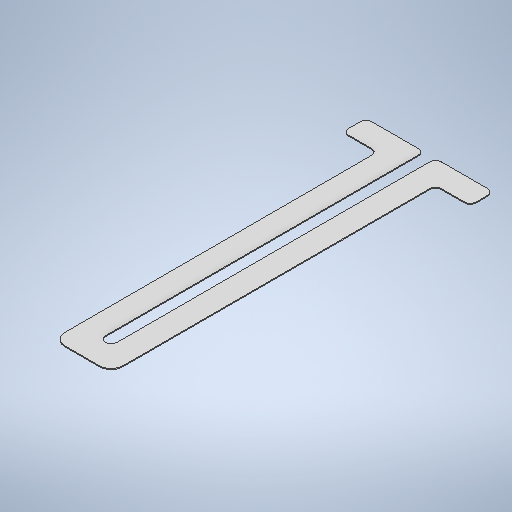
# Autodesk Inventor part: Medio
Saved by Autodesk Inventor 2025.4 (Build 294407000, 407)
## iProperties
Created: 2026-04-15
Part Number: Medio
Material: Generic
Document SubType Name: Modeling
Designer: gdira
Density: 1 g/cm^3
Appearance: Default
Author: gdira
Autodesk Inventor part; units mm, degrees
ref_plane "YZ Plane" through (0, 0, 0) normal (1, 0, 0) x (0, 1, 0)
ref_plane "XZ Plane" through (0, 0, 0) normal (0, 1, 0) x (-1, 0, 0)
ref_plane "XY Plane" through (0, 0, 0) normal (0, 0, 1) x (1, 0, 0)
sketch "Sketch1" plane through (0, 0, 0) normal (0, 1, 0) x (-1, 0, 0)
  line L0 (1.2188, -16.0155) -> (-0.7718, -16.0155)
  line L1 (-4.7718, -16.0123) -> (-12.7718, -16.0123)
  line L2 (1.2188, -16.0155) -> (7.23, -16.0045)
  line L3 (-3.7718, 38.99) -> (-3.7718, -15.0123)
  line L4 (-1.7718, -15.0155) -> (-1.7718, 38.99)
  line L5 (-2.7718, 39.99) -> (-2.7718, 39.99)
  line L6 (-7.7718, 41.99) -> (-7.7718, -8.0123)
  line L7 (-5.7718, 43.99) -> (0.2282, 43.99)
  line L8 (2.2282, 41.99) -> (2.2282, -7.9845)
  arc A0 (-5.7718, 43.99) -> (-7.7718, 41.99) centre (-5.7718, 41.99) ccw
  arc A1 (2.2282, 41.99) -> (0.2282, 43.99) centre (0.2282, 41.99) ccw
  line L9 (8.2282, -15.0045) -> (8.2282, -13.0027)
  line L10 (7.2282, -12.0027) -> (3.2282, -12.0027)
  line L11 (2.2282, -11.0027) -> (2.2282, -4.4303)
  line L12 (-13.7718, -15.0123) -> (-13.7718, -13.0123)
  line L13 (-12.7718, -12.0123) -> (-8.7718, -12.0123)
  line L14 (-7.7718, -11.0123) -> (-7.7718, -8.0123)
  arc A2 (-8.7718, -12.0123) -> (-7.7718, -11.0123) centre (-8.7718, -11.0123) ccw
  arc A3 (-12.7718, -12.0123) -> (-13.7718, -13.0123) centre (-12.7718, -13.0123) ccw
  arc A4 (-13.7718, -15.0123) -> (-12.7718, -16.0123) centre (-12.7718, -15.0123) ccw
  arc A5 (-4.7718, -16.0123) -> (-3.7718, -15.0123) centre (-4.7718, -15.0123) ccw
  arc A6 (-1.7718, -15.0155) -> (-0.7718, -16.0155) centre (-0.7718, -15.0155) ccw
  arc A7 (7.23, -16.0045) -> (8.2282, -15.0045) centre (7.2282, -15.0045) ccw
  arc A8 (8.2282, -13.0027) -> (7.2282, -12.0027) centre (7.2282, -13.0027) ccw
  arc A9 (2.2282, -11.0027) -> (3.2282, -12.0027) centre (3.2282, -11.0027) ccw
  arc A10 (-2.7718, 39.99) -> (-3.7718, 38.99) centre (-2.7718, 38.99) ccw
  arc A11 (-1.7718, 38.99) -> (-2.7718, 39.99) centre (-2.7718, 38.99) ccw
  point P0 (0, 0)
  point P1 (1.9085, 4.4205)
  point P2 (-1.7718, -16.0155)
  point P3 (4.2244, -16.01)
  point P4 (-13.7718, -16.0123)
  point P5 (8.2282, -16.0027)
  point P6 (-2.7718, 39.99)
  point P7 (-2.7718, 43.99)
  point P8 (8.2282, -12.0027)
  point P9 (-13.7718, -12.0123)
  point P10 (-2.7718, 39.99)
  dimension "d0" = 10
  dimension "d1" = 4
  dimension "d2" = 4
  dimension "d3" = 2
  dimension "d4" = 4
  dimension "d5" = 60
  dimension "d6" = 2
  dimension "d7" = 4
  dimension "d8" = 4
  dimension "d9" = 1
  dimension "d10" = 1
  constraints: 30 end point, 24 point on circle, 24 tangent, 12 centre point, 11 point on line, 9 equal radius, 5 perpendicular, 3 midpoint, 2 horizontal, 2 vertical, 1 collinear, 1 parallel
  measures "d0" distance of point (8.228, -16.003) point (-1.772, -16.015)
  measures "d1" distance between parallel lines of L4 L8
  measures "d2" distance between parallel lines of L6 L3
  measures "d3" distance between parallel lines of L3 L4
  measures "d4" distance of point (-2.772, 43.99) point (-2.772, 39.99)
  measures "d5" distance from line of point (4.224, -16.01) L7
  measures "d6" radius of A0
  measures "d7" distance of point (8.228, -16.003) point (8.228, -12.003)
  measures "d8" distance of point (-13.772, -16.012) point (-13.772, -12.012)
  measures "d9" radius of A2
  measures "d10" radius of A10
extrude "Extrusion1" add sketch "Sketch1" along normal blind 0.15
body "Solid1"
